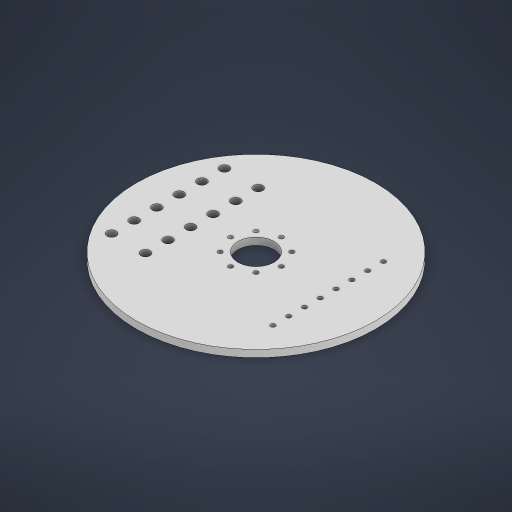
# Autodesk Inventor part: ArmBase
Saved by Autodesk Inventor 2024 (Build 280153000, 153)
## iProperties
Created: 2024-01-05
Part Number: ArmBase
Material: Generic
Document SubType Name: Modeling
Designer: avsar
Density: 1 g/cm^3
Appearance: Default
Author: avsar
Autodesk Inventor part; units mm, degrees
ref_plane "YZ Plane" through (0, 0, 0) normal (1, 0, 0) x (0, 1, 0)
ref_plane "XZ Plane" through (0, 0, 0) normal (0, 1, 0) x (-1, 0, 0)
ref_plane "XY Plane" through (0, 0, 0) normal (0, 0, 1) x (1, 0, 0)
sketch "Sketch1" plane through (0, 0, 0) normal (0, 1, 0) x (-1, 0, 0)
  circle A0 centre (0, 0) radius 106
  dimension "d1" = 212
  constraints: 1 centre point, 1 coincident
  measures "d1" diameter of A0
extrude "Extrusion1" add sketch "Sketch1" along normal mid plane 6.35
sketch "Sketch2" plane through (0, 3.175, 0) normal (0, 1, 0) x (1, 0, 0)
  circle A0 centre (0, 22.5) radius 2.05
  circle A1 centre (-15.9099, 15.9099) radius 2.05
  circle A2 centre (-22.5, 0) radius 2.05
  circle A3 centre (-15.9099, -15.9099) radius 2.05
  circle A4 centre (0, -22.5) radius 2.05
  circle A5 centre (15.9099, -15.9099) radius 2.05
  circle A6 centre (22.5, 0) radius 2.05
  circle A7 centre (15.9099, 15.9099) radius 2.05
  point P0 (0, 0)
  dimension "d4" = 4.1
  dimension "d5" = 22.5
  dimension "d8" = 360
  constraints: 8 centre point, 1 vertical alignment, 17 other
  measures "d4" diameter of A0
  measures "d5" distance of point (0, 0) A0.centre
extrude "Extrusion2" cut sketch "Sketch2" against normal through all
sketch "Sketch3" plane through (0, 3.175, 0) normal (0, 1, 0) x (1, 0, 0)
  circle A0 centre (0, 0) radius 16.1
  dimension "d12" = 32.2
  constraints: 1 centre point, 1 coincident
  measures "d12" diameter of A0
extrude "Extrusion3" cut sketch "Sketch3" against normal through all
sketch "Sketch4" plane through (0, 3.175, 0) normal (0, 1, 0) x (1, 0, 0)
  circle A0 centre (-48, -50) radius 4.1
  circle A1 centre (0, 0) radius 16.1 construction
  line L0 (0, -16.1) -> (0, 16.1) construction
  circle A2 centre (-48, -30) radius 4.1
  circle A3 centre (-48, -10) radius 4.1
  circle A4 centre (-48, 10) radius 4.1
  circle A5 centre (-48, 30) radius 4.1
  circle A6 centre (-48, 50) radius 4.1
  line L1 (-16.1, 0) -> (16.1, 0)
  circle A7 centre (-78, -10) radius 4.1
  circle A8 centre (-78, 10) radius 4.1
  circle A9 centre (-78, -30) radius 4.1
  circle A10 centre (-78, 30) radius 4.1
  circle A11 centre (-78, -50) radius 4.1
  circle A12 centre (-78, 50) radius 4.1
  dimension "d15" = 8.2
  dimension "d16" = 50
  dimension "d17" = 48
  dimension "d20" = 20
  dimension "d36" = 30
  constraints: 12 centre point, 4 end point, 4 point on circle, 2 horizontal, 2 midpoint, 2 vertical, 1 coincident, 22 other
  measures "d15" diameter of A0
  measures "d16" vertical distance of point (0, 0) A0.centre
  measures "d17" horizontal distance of point (0, 0) A0.centre
  measures "d20" distance of A0.centre A2.centre
  measures "d36" distance of A3.centre A7.centre
extrude "Extrusion4" cut sketch "Sketch4" against normal through all
sketch "Sketch6" plane through (0, 3.175, 0) normal (0, 1, 0) x (1, 0, 0)
  circle A0 centre (-48, -50) radius 4.1 construction
  circle A1 centre (64, -49) radius 2.1
  circle A2 centre (0, 0) radius 16.1 construction
  line L0 (0, 16.1) -> (0, -16.1) construction
  circle A3 centre (64, -35) radius 2.1
  circle A4 centre (64, -21) radius 2.1
  circle A5 centre (64, -7) radius 2.1
  circle A6 centre (64, 7) radius 2.1
  circle A7 centre (64, 21) radius 2.1
  circle A8 centre (64, 35) radius 2.1
  circle A9 centre (64, 49) radius 2.1
  line L1 (64, -7) -> (64, 7) construction
  point P0 (64, 0)
  dimension "d41" = 4.2
  dimension "d42" = 64
  dimension "d45" = 14
  constraints: 8 centre point, 4 end point, 3 vertical, 2 midpoint, 2 point on circle, 1 coincident, 1 horizontal alignment, 14 other
  measures "d41" diameter of A1
  measures "d42" horizontal distance of point (0, 0) A1.centre
  measures "d45" distance of A1.centre A3.centre
extrude "Extrusion5" cut sketch "Sketch6" against normal through all
body "Solid1"
